Autodesk Inventor part; units mm, degrees
(part 2 of 2)
sketch "Sketch10" plane through (0, 0, 9.3) normal (0, 0, 1) x (1, 0, 0)
  arc A0 (3, -24.6) -> (1.5, -23.1) centre (1.5, -24.6) ccw construction
  line L0 (0, -23.1) -> (1.5, -23.1) construction
  line L1 (0, -33.0895) -> (0, -23.1) construction
  spline S0 degree 2 poles (0, -33.0895) (1.5718, -35.1685) (0, -37.2476) knots 0 0 0 1 1 1 weights 1 1.527778 1 construction
  line L2 (0, -41.3315) -> (0, -37.2476) construction
  line L3 (3, -24.6) -> (3, -29.7467) construction
  circle A1 centre (20.3345, -9.75) radius 2.25
  line L4 (8.9062, -65.3371) -> (8.9062, -65.8371)
  line L5 (13.0938, -65.8371) -> (8.9062, -65.8371)
  line L6 (13.0938, -65.8371) -> (13.0938, -65.3371)
  line L7 (13.0938, -65.3371) -> (15.9062, -65.3371)
  line L8 (15.9062, -65.3371) -> (15.9062, -65.8371)
  line L9 (23.1, -65.8371) -> (15.9062, -65.8371)
  line L10 (23.1, -6.5) -> (23.1, -65.8371)
  line L11 (27.4, -6.5) -> (23.1, -6.5)
  line L12 (27.4, 0) -> (27.4, -6.5)
  line L13 (0, 0) -> (27.4, 0)
  line L14 (0, -3.5) -> (0, 0)
  line L15 (1, -3.5) -> (0, -3.5)
  line L16 (1, -1) -> (1, -3.5)
  line L17 (2.5, -1) -> (1, -1)
  line L18 (2.5, -17.5) -> (2.5, -1)
  line L19 (1, -17.5) -> (2.5, -17.5)
  line L20 (1, -15) -> (1, -17.5)
  line L21 (0, -15) -> (1, -15)
  line L22 (0, -65.8371) -> (0, -15)
  line L23 (6.0938, -65.8371) -> (0, -65.8371)
  line L24 (6.0938, -65.8371) -> (6.0938, -65.3371)
  line L25 (6.0938, -65.3371) -> (8.9062, -65.3371)
  circle A2 centre (7.5, -9.75) radius 3
  circle A3 centre (14, -49.1746) radius 3
  circle A4 centre (17.6, -58.8371) radius 3
  circle A5 centre (3.5, -62.3371) radius 3
  circle A6 centre (4, -46.5095) radius 3
  arc A7 (19.4959, -28.2768) -> (17.618, -23.3446) centre (19.8907, -25.3029) ccw
  arc A8 (4.0542, -29.6883) -> (19.4959, -28.2768) centre (12.35, -35.2722) ccw
  arc A9 (9.7, -14.6801) -> (4.0542, -29.6883) centre (9.2226, -23.0665) ccw
  arc A10 (16.7181, -19.2746) -> (9.7, -14.6801) centre (14.7, -14.7) ccw
  arc A11 (17.618, -23.3446) -> (16.7181, -19.2746) centre (9.2226, -23.0665) ccw
  circle A12 centre (1.5356, -30.0714) radius 1
  circle A13 centre (1.5, -41.3315) radius 1
  circle A14 centre (1.5356, -30.0714) radius 2
  circle A15 centre (1.5, -41.3315) radius 2
  circle A16 centre (4, -46.5095) radius 3.5
  arc A17 (4.0542, -29.6883) -> (19.4959, -28.2768) centre (12.35, -35.2722) ccw
  arc A18 (9.7, -14.6801) -> (4.0542, -29.6883) centre (9.2226, -23.0665) ccw
  circle A19 centre (1.5, -41.3315) radius 2.25
  arc A20 (3, -41.3315) -> (0, -41.3315) centre (1.5, -41.3315) ccw
  line L26 (3, -30.3961) -> (3, -41.3315)
  arc A21 (3, -29.7467) -> (3, -30.3961) centre (1.5356, -30.0714) ccw
  point P0 (0, 0)
  dimension "d145" = 2
  dimension "d146" = 2
  dimension "d147" = 4
  dimension "d148" = 4
  dimension "d149" = 7
  dimension "d150" = 1.5
  dimension "d151" = 1.5
  dimension "d152" = 4.5
  constraints: 6 centre point, 4 coincident, 3 tangent
  measures "d145" diameter of A12
  measures "d146" diameter of A13
  measures "d147" diameter of A14
  measures "d148" diameter of A15
  measures "d149" diameter of A16
  measures "d150" distance from line of L3 A13.centre
  measures "d151" distance from line of L2 A13.centre
  measures "d152" diameter of A19
hole "Hole7" at (1.5356, -30.0714, 9.3) at (1.5, -41.3315, 9.3) direction (0, 0, -1) diameter 2 end through all clearance for "Countersunk Flat Head Screw ISO 2009/7046" size "M2" standard "ISO"
body "Solid2"
